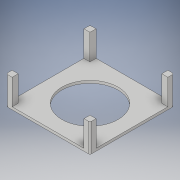
# Autodesk Inventor part: suporte interno
Saved by Autodesk Inventor 2019.4 (Build 234330000, 330)
## iProperties
Created: 2019-11-28
Part Number: suporte interno
Material: Genérico
Document SubType Name: Modeling
Designer: natha
Density: 1 g/cm^3
Appearance: Padrão
Author: natha
Autodesk Inventor part; units mm, degrees
ref_plane "YZ Plane" through (0, 0, 0) normal (1, 0, 0) x (0, 1, 0)
ref_plane "XZ Plane" through (0, 0, 0) normal (0, 1, 0) x (-1, 0, 0)
ref_plane "XY Plane" through (0, 0, 0) normal (0, 0, 1) x (1, 0, 0)
sketch "Esboço1" plane through (0, 0, 0) normal (0, 1, 0) x (-1, 0, 0)
  line L0 (-46.5, 48.5) -> (46.5, 48.5)
  line L1 (48.5, 46.5) -> (48.5, -46.5)
  line L2 (46.5, -48.5) -> (-46.5, -48.5)
  line L3 (-48.5, -46.5) -> (-48.5, 46.5)
  line L4 (-48.5, 48.5) -> (48.5, -48.5) construction
  line L5 (48.5, 48.5) -> (-48.5, -48.5) construction
  arc A0 (48.5, 46.5) -> (46.5, 48.5) centre (46.5, 46.5) ccw
  arc A1 (-46.5, 48.5) -> (-48.5, 46.5) centre (-46.5, 46.5) ccw
  arc A2 (-48.5, -46.5) -> (-46.5, -48.5) centre (-46.5, -46.5) ccw
  arc A3 (46.5, -48.5) -> (48.5, -46.5) centre (46.5, -46.5) ccw
  point P0 (0, 0)
  dimension "d0" = 97
  dimension "d1" = 97
  dimension "d2" = 2
  constraints: 12 end point, 8 point on circle, 8 point on line, 8 tangent, 4 centre point, 3 equal radius, 2 midpoint, 2 parallel, 1 horizontal, 1 perpendicular
  measures "d0" distance of L4.end L5.end
  measures "d1" distance of L5.end L4.start
  measures "d2" radius of A0
extrude "Extrusão1" add sketch "Esboço1" along normal blind 3
sketch "Esboço2" plane through (0, 3, 0) normal (0, 1, 0) x (1, 0, 0)
  line L0 (-46.5, -48.5) -> (46.5, -48.5) projected
  arc A0 (46.5, -48.5) -> (48.5, -46.5) centre (46.5, -46.5) ccw projected
  line L1 (48.5, -46.5) -> (48.5, 46.5) projected
  arc A1 (48.5, 46.5) -> (46.5, 48.5) centre (46.5, 46.5) ccw projected
  line L2 (46.5, 48.5) -> (-46.5, 48.5) projected
  arc A2 (-46.5, 48.5) -> (-48.5, 46.5) centre (-46.5, 46.5) ccw projected
  line L3 (-48.5, 46.5) -> (-48.5, -46.5) projected
  arc A3 (-48.5, -46.5) -> (-46.5, -48.5) centre (-46.5, -46.5) ccw projected
  line L4 (-46.5, -48.5) -> (-41.5, -48.5)
  line L5 (-41.5, -48.5) -> (-41.5, -41.5)
  line L6 (-41.5, -41.5) -> (-48.5, -41.5)
  line L7 (-48.5, -41.5) -> (-48.5, -46.5)
  line L8 (-46.5, 48.5) -> (-41.5, 48.5)
  line L9 (-41.5, 48.5) -> (-41.5, 41.5)
  line L10 (-41.5, 41.5) -> (-48.5, 41.5)
  line L11 (-48.5, 41.5) -> (-48.5, 46.5)
  line L12 (46.5, -48.5) -> (41.5, -48.5)
  line L13 (41.5, -48.5) -> (41.5, -41.5)
  line L14 (41.5, -41.5) -> (48.5, -41.5)
  line L15 (48.5, -41.5) -> (48.5, -46.5)
  line L16 (46.5, 48.5) -> (41.5, 48.5)
  line L17 (41.5, 48.5) -> (41.5, 41.5)
  line L18 (41.5, 41.5) -> (48.5, 41.5)
  line L19 (48.5, 41.5) -> (48.5, 46.5)
  arc A4 (-48.5, -46.5) -> (-46.5, -48.5) centre (-46.5, -46.5) ccw
  arc A5 (-46.5, 48.5) -> (-48.5, 46.5) centre (-46.5, 46.5) ccw
  arc A6 (48.5, 46.5) -> (46.5, 48.5) centre (46.5, 46.5) ccw
  arc A7 (46.5, -48.5) -> (48.5, -46.5) centre (46.5, -46.5) ccw
  point P0 (0, 0)
  point P1 (-48.5, -48.5)
  point P2 (48.5, 48.5)
  dimension "d6" = 7
  dimension "d7" = 7
  dimension "d8" = 7
  dimension "d9" = 7
  dimension "d10" = 7
  dimension "d11" = 7
  dimension "d12" = 7
  dimension "d13" = 7
  dimension "d14" = 2
  constraints: 32 end point, 8 parallel, 8 point on circle, 8 tangent, 7 point on line, 4 centre point, 4 horizontal, 4 perpendicular, 3 equal radius
  measures "d6" distance of L6.end L5.end
  measures "d7" distance of L4.end L5.end
  measures "d8" distance of L9.end L10.end
  measures "d9" distance of L8.end L9.end
  measures "d10" distance of L13.end L14.end
  measures "d11" distance of L12.end L13.end
  measures "d12" distance of L18.end L17.end
  measures "d13" distance of L17.end L16.end
  measures "d14" radius of A4
sketch "Esboço3" plane through (0, 0, 0) normal (0, -1, 0) x (1, 0, 0)
  circle A0 centre (0, 0) radius 32.5
  dimension "d15" = 65
  constraints: 1 centre point, 1 coincident
  measures "d15" diameter of A0
extrude "Extrusão2" cut sketch "Esboço3" against normal blind 3
extrude "Extrusão3" add sketch "Esboço2" along normal blind 29.6 contours A3 L3 L6 L5 L0 | L13 L14 L1 A0 L0 | L3 A2 L2 L9 L10 | L18 L17 L2 A1 L1
